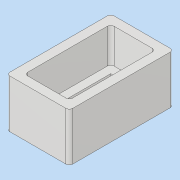
# Autodesk Inventor part: ForeConnectorHousing
Saved by Autodesk Inventor 2017 (Build 210142000, 142)
## iProperties
Created: 2019-07-18
Part Number: ForeConnectorHousing
Material: ABS Plastic
Document SubType Name: Modeling
Designer: techn
Density: 1.06 g/cm^3
Appearance: Smooth - White
Author: techn
Autodesk Inventor part; units mm, degrees
ref_plane "YZ Plane" through (0, 0, 0) normal (1, 0, 0) x (0, 1, 0)
ref_plane "XZ Plane" through (0, 0, 0) normal (0, 1, 0) x (-1, 0, 0)
ref_plane "XY Plane" through (0, 0, 0) normal (0, 0, 1) x (1, 0, 0)
sketch "Sketch1" plane through (0, 0, 0) normal (0, 1, 0) x (-1, 0, 0)
  line L0 (0, 0) -> (11.557, 0)
  line L1 (11.557, 0) -> (11.557, -19.177)
  line L2 (11.557, -19.177) -> (0, -19.177)
  line L3 (0, -19.177) -> (0, 0)
  line L4 (3.175, -3.175) -> (8.382, -3.175)
  line L5 (8.382, -3.175) -> (8.382, -16.002)
  line L6 (8.382, -16.002) -> (3.175, -16.002)
  line L7 (3.175, -16.002) -> (3.175, -3.175)
  line L8 (8.382, -3.175) -> (5.969, -3.175)
  line L9 (5.969, -3.175) -> (5.969, -5.588)
  line L10 (5.969, -5.588) -> (8.382, -5.588)
  line L11 (8.382, -5.588) -> (8.382, -3.175)
  dimension "d0" = 12.827
  dimension "d1" = 5.207
  dimension "d2" = 3.175
  dimension "d3" = 3.175
  dimension "d4" = 3.175
  dimension "d5" = 3.175
  dimension "d6" = 2.413
  dimension "d7" = 2.413
  constraints: 24 end point, 6 parallel, 3 horizontal, 3 perpendicular
  measures "d0" distance of L6.end L4.start
  measures "d1" distance of L5.end L6.end
  measures "d2" distance between parallel lines of L0 L4
  measures "d3" distance between parallel lines of L2 L6
  measures "d4" distance between parallel lines of L1 L5
  measures "d5" distance between parallel lines of L7 L3
  measures "d6" distance of L10.end L9.end
  measures "d7" distance of L9.end L8.end
extrude "Extrusion1" add sketch "Sketch1" along normal blind 2.54 contours L0 L1 L2 L3 | L4 L5 L10 L9
sketch "Sketch2" plane through (0, 2.54, 0) normal (0, 1, 0) x (1, 0, 0)
  line L0 (-8.382, 5.588) -> (-8.382, 16.002) construction
  line L1 (-8.382, 16.002) -> (-3.175, 16.002) construction
  line L2 (-3.175, 16.002) -> (-3.175, 3.175) construction
  line L3 (-3.175, 3.175) -> (-5.969, 3.175) construction
  line L4 (-5.969, 3.175) -> (-5.969, 5.588) construction
  line L5 (-5.969, 5.588) -> (-8.382, 5.588) construction
  line L6 (-11.557, 19.177) -> (-11.557, 0) projected
  line L7 (-11.557, 0) -> (0, 0) projected
  line L8 (0, 0) -> (0, 19.177) projected
  line L9 (0, 19.177) -> (-11.557, 19.177) projected
  line L10 (-9.906, 1.651) -> (-1.651, 1.651)
  line L11 (-1.651, 1.651) -> (-1.651, 17.526)
  line L12 (-1.651, 17.526) -> (-9.906, 17.526)
  line L13 (-9.906, 17.526) -> (-9.906, 1.651)
  dimension "d10" = 1.524
  dimension "d11" = 1.524
  dimension "d14" = 1.524
  dimension "d15" = 1.524
  constraints: 8 end point, 2 parallel, 1 horizontal, 1 perpendicular
  measures "d10" distance between parallel lines of L13 L0
  measures "d11" distance between parallel lines of L10 L3
  measures "d14" distance between parallel lines of L11 L2
  measures "d15" distance between parallel lines of L12 L1
extrude "Extrusion2" add sketch "Sketch2" along normal blind 6.35
fillet "Fillet1" radius 0.635 8 edges at (0, 4.445, 0) (-11.557, 4.445, 0) (-11.557, 4.445, -19.177) (0, 4.445, -19.177) (-9.906, 5.715, -17.526) (-9.906, 5.715, -1.651) (-1.651, 5.715, -17.526) (-1.651, 5.715, -1.651)
equation "\"d3\" = d2"
equation "\"d4\" = d2"
equation "\"d5\" = d4"
equation "\"d11\" = d10"
equation "\"d14\" = d10"
equation "\"d15\" = d10"
body "Solid1"
